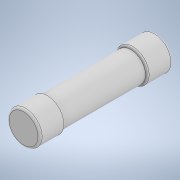
# Autodesk Inventor part: Fusible de 13A
Saved by Autodesk Inventor 2021 (Build 250183000, 183)
## iProperties
Created: 2021-05-26
Part Number: Fusible de 13A
Material: Generic
Document SubType Name: Modeling
Designer: Nelson
Density: 14.7595 g/cm^3
Appearance: Default
Mass: 10 g
Surface Area: 5.2381 cm^2
Volume: 0.677532 cm^3
Author: Nelson
Autodesk Inventor part; units mm, degrees
ref_plane "YZ Plane" through (0, 0, 0) normal (1, 0, 0) x (0, 1, 0)
ref_plane "XZ Plane" through (0, 0, 0) normal (0, 1, 0) x (-1, 0, 0)
ref_plane "XY Plane" through (0, 0, 0) normal (0, 0, 1) x (1, 0, 0)
sketch "Sketch2" plane through (0, 0, 0) normal (1, 0, 0) x (0, 1, 0)
  line L0 (0, 0) -> (3.15, 0)
  line L1 (3.15, 0) -> (3.15, -4.9)
  line L2 (3.15, -4.9) -> (2.8, -4.9)
  line L3 (2.8, -4.9) -> (2.8, -20.5)
  line L4 (2.8, -20.5) -> (3.15, -20.5)
  line L5 (3.15, -20.5) -> (3.15, -25.4)
  line L6 (3.15, -25.4) -> (0, -25.4)
  line L7 (0, -25.4) -> (0, 0)
  dimension "d1" = 3.15
  dimension "d2" = 4.9
  dimension "d3" = 0.35
  dimension "d4" = 15.6
  dimension "d5" = 0.35
  dimension "d6" = 4.9
  dimension "d7" = 3.15
  constraints: 16 end point, 3 perpendicular, 2 point on line, 1 horizontal, 1 vertical
  measures "d1" distance of L0.start L0.end
  measures "d2" distance of L0.end L1.end
  measures "d3" distance of L1.end L2.end
  measures "d4" distance of L2.end L3.end
  measures "d5" distance of L3.end L4.end
  measures "d6" distance of L4.end L5.end
  measures "d7" distance of L5.end L6.end
revolve "Revolution1" add sketch "Sketch2" angle 360 about axis through (0, 0, -25.4) along (0, 0, 1)
fillet "Fillet4" radius 0.4 2 edges at (0, -3.15, -25.4) (0, -3.15, 0)
fillet "Fillet5" radius 0.35 2 edges at (0, -3.15, -20.5) (0, -3.15, -4.9)
equation "\"d5\" = d3"
equation "\"d6\" = d2"
equation "\"d7\" = d1"
body "Solid1"
